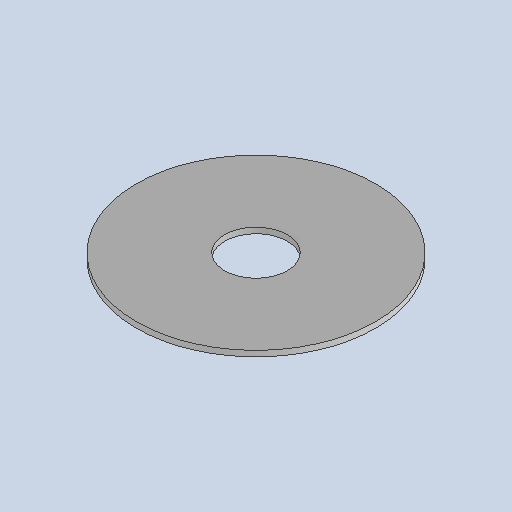
# Autodesk Inventor part: ДМС 040 лицо крышка
Saved by Autodesk Inventor 2024.2 (Build 282272000, 272)
## iProperties
Created: 2024-04-23
Part Number: ДМС 040 лицо крышка
Material: Generic
Document SubType Name: Modeling
Designer: admin
Density: 1 g/cm^3
Appearance: Default
Author: admin
Autodesk Inventor part; units mm, degrees
ref_plane "YZ Plane" through (0, 0, 0) normal (1, 0, 0) x (0, 1, 0)
ref_plane "XZ Plane" through (0, 0, 0) normal (0, 1, 0) x (-1, 0, 0)
ref_plane "XY Plane" through (0, 0, 0) normal (0, 0, 1) x (1, 0, 0)
sketch "Sketch1" plane through (0, 0, 0) normal (0, 0, 1) x (1, 0, 0)
  circle A0 centre (0, 0) radius 200 construction
  circle A1 centre (0, 0) radius 210
  circle A2 centre (0, 0) radius 55
  dimension "d0" = 400
  dimension "d4" = 110
  dimension "d13" = 10
  constraints: 3 centre point, 3 coincident
  measures "d0" diameter of A0
  measures "d4" diameter of A2
  measures "d13" radial gap between concentric circles of A1 A0
extrude "Extrusion1" add sketch "Sketch1" along normal blind 10
equation "\"d0\" = Шпил_пласт_НОС_диам_центров"
equation "\"d4\" = Диам_отв_крышка_грязи"
equation "\"Шпил_пласт_НОС_диам_центров\" = 400"
equation "\"Диам_отв_крышка_грязи\" = 110"
body "Solid1"
